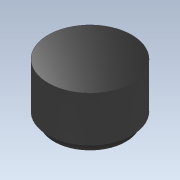
# Autodesk Inventor part: Speakertje
Saved by Autodesk Inventor 2020.3 (Build 243373000, 373)
## iProperties
Created: 2020-10-24
Part Number: Speakertje
Material: Generic
Document SubType Name: Modeling
Designer: Britt
Density: 1 g/cm^3
Appearance: Glossy - Black
Author: Britt
Autodesk Inventor part; units mm, degrees
ref_plane "YZ Plane" through (0, 0, 0) normal (1, 0, 0) x (0, 1, 0)
ref_plane "XZ Plane" through (0, 0, 0) normal (0, 1, 0) x (-1, 0, 0)
ref_plane "XY Plane" through (0, 0, 0) normal (0, 0, 1) x (1, 0, 0)
sketch "Sketch1" plane through (0, 0, 0) normal (0, 0, 1) x (1, 0, 0)
  line L0 (0, 0) -> (0, 45)
  line L1 (0, 45) -> (35, 45)
  line L2 (35, 45) -> (35, 7)
  line L3 (35, 7) -> (30, 7)
  line L4 (30, 7) -> (30, 0)
  line L5 (30, 0) -> (0, 0)
  dimension "d0" = 45
  dimension "d1" = 35
  dimension "d2" = 38
  dimension "d3" = 5
  constraints: 12 end point, 5 perpendicular, 1 vertical
  measures "d0" distance of L0.start L0.end
  measures "d1" distance of L0.end L1.end
  measures "d2" distance of L1.end L2.end
  measures "d3" distance of L2.end L3.end
revolve "Revolution1" add sketch "Sketch1" angle 360 about axis through (0, 0, 0) along (0, 1, 0)
body "Solid1"
